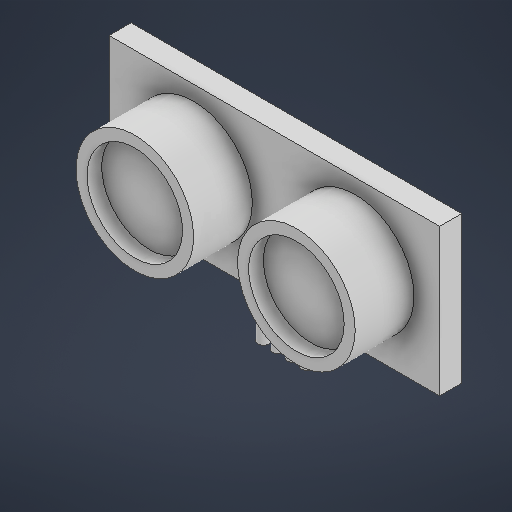
# Autodesk Inventor part: US HC-SR04
Saved by Autodesk Inventor 2026.2 (Build 302298010, 298A)
## iProperties
Created: 2026-03-17
Part Number: US HC-SR04
Material: Générique
Document SubType Name: Modeling
Designer: cleml
Density: 1 g/cm^3
Appearance: Par défaut
Author: cleml
Autodesk Inventor part; units mm, degrees
ref_plane "YZ Plane" through (0, 0, 0) normal (1, 0, 0) x (0, 1, 0)
ref_plane "XZ Plane" through (0, 0, 0) normal (0, 1, 0) x (-1, 0, 0)
ref_plane "XY Plane" through (0, 0, 0) normal (0, 0, 1) x (1, 0, 0)
sketch "Esquisse1" plane through (0, 0, 0) normal (0, 0, 1) x (1, 0, 0)
  line L0 (0, 0) -> (45, 0)
  line L1 (45, 0) -> (45, 20)
  line L2 (45, 20) -> (0, 20)
  line L3 (0, 20) -> (0, 0)
  dimension "d0" = 45
  dimension "d1" = 20
  constraints: 8 end point, 2 parallel, 1 horizontal, 1 perpendicular
  measures "d0" distance of L1.end L2.end
  measures "d1" distance of L0.end L1.end
extrude "Extrusion1" add sketch "Esquisse1" along normal blind 3
sketch "Esquisse2" plane through (0, 0, 3) normal (0, 0, 1) x (1, 0, 0)
  line L0 (45, 0) -> (45, 20) projected
  line L1 (0, 0) -> (45, 0) projected
  circle A0 centre (11.5, 10) radius 8
  circle A1 centre (33.5, 10) radius 8
  dimension "d4" = 22
  dimension "d5" = 11.5
  dimension "d6" = 10
  dimension "d7" = 10
  dimension "d8" = 16
  dimension "d9" = 16
  constraints: 2 centre point, 2 coincident
  measures "d4" distance of point (33.5, 10) point (11.5, 10)
  measures "d5" distance from line of L0 point (33.5, 10)
  measures "d6" distance from line of L1 point (33.5, 10)
  measures "d7" distance from line of L1 point (11.5, 10)
  measures "d8" diameter of A0
  measures "d9" diameter of A1
extrude "Extrusion2" add sketch "Esquisse2" along normal blind 8
sketch "Esquisse3" plane through (11.5, 10, 11) normal (0, 0, 1) x (1, 0, 0)
  circle A0 centre (0, 0) radius 6.5
  circle A1 centre (22, 0) radius 8 projected
  circle A2 centre (22, 0) radius 6.5
  circle A3 centre (0, 0) radius 7.9442
  circle A4 centre (22, 0) radius 8
  point P0 (-11.5, -10)
  dimension "d12" = 13
  dimension "d13" = 13
  constraints: 4 centre point, 3 coincident, 1 concentric
  measures "d12" diameter of A0
  measures "d13" diameter of A2
extrude "Extrusion3" cut sketch "Esquisse3" against normal blind 2 contours A0 | A2
sketch "Esquisse4" plane through (0, 0, 0) normal (0, -1, 0) x (1, 0, 0)
  line L0 (45, 0) -> (45, 3) projected
  circle A0 centre (19.5, 1.5) radius 0.75
  circle A1 centre (21.5, 1.5) radius 0.75
  circle A2 centre (23.5, 1.5) radius 0.75
  circle A3 centre (25.5, 1.5) radius 0.75
  line L1 (0, 3) -> (45, 3) projected
  point P0 (0, 0)
  dimension "d17" = 2
  dimension "d18" = 2
  dimension "d19" = 2
  dimension "d22" = 1.5
  dimension "d23" = 1.5
  dimension "d24" = 1.5
  dimension "d25" = 1.5
  dimension "d26" = 19.5
  dimension "d29" = 1.5
  dimension "d30" = 3
  constraints: 4 centre point, 4 coincident
  measures "d17" distance of point (21.5, 1.5) point (19.5, 1.5)
  measures "d18" distance of point (23.5, 1.5) point (21.5, 1.5)
  measures "d19" distance of point (23.5, 1.5) point (25.5, 1.5)
  measures "d22" diameter of A0
  measures "d23" diameter of A1
  measures "d24" diameter of A2
  measures "d25" diameter of A3
  measures "d26" distance from line of L0 point (25.5, 1.5)
  measures "d29" distance from line of L1 point (25.5, 1.5)
  measures "d30" distance of L0.start L0.end
extrude "Extrusion4" add sketch "Esquisse4" along normal blind 7
equation "\"d7\" = d6"
equation "\"d18\" = d17"
equation "\"d19\" = d17"
equation "\"d29\" = 0.5 * d30"
